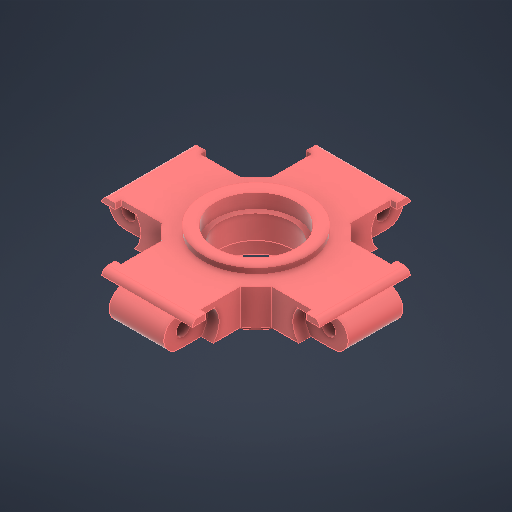
# Autodesk Inventor part: SujeccionHelices
Saved by Autodesk Inventor 2026.1 (Build 301233000, 233)
## iProperties
Created: 2025-11-10
Part Number: SujeccionHelices
Material: PLA
Document SubType Name: Modeling
Designer: vickh
Density: 1.3 g/cm^3
Appearance: Suave - Rojo
Mass: 57.6997 g
Surface Area: 138.679 cm^2
Volume: 44.3844 cm^3
Author: vickh
## iProperties of the stored document SujeccionHelices_3DPrint.ipt
Created: 2025-11-17
Part Number: SujeccionHelices_3DPrint
Material: Genérico
Document SubType Name: Modeling
Designer: usuario
Density: 1 g/cm^3
Appearance: Valor por defecto
Author: usuario
Autodesk Inventor part; units mm, degrees
ref_plane "YZ Plane" through (0, 0, 0) normal (1, 0, 0) x (0, 1, 0)
ref_plane "XZ Plane" through (0, 0, 0) normal (0, 1, 0) x (-1, 0, 0)
ref_plane "XY Plane" through (0, 0, 0) normal (0, 0, 1) x (1, 0, 0)
sketch "Boceto27" plane through (0, 0, 0) normal (0, 1, 0) x (-1, 0, 0)
  line L0 (13.15, -40) -> (-13.15, -40)
  line L1 (-13.15, 40) -> (13.15, 40)
  line L2 (13.15, 40) -> (-13.15, -40) construction
  line L3 (13.15, -40) -> (-13.15, 40) construction
  line L4 (-40, 13.15) -> (-40, -13.15)
  line L5 (40, -13.15) -> (40, 13.15)
  line L6 (-40, 13.15) -> (40, -13.15) construction
  line L7 (-40, -13.15) -> (40, 13.15) construction
  line L8 (40, 13.15) -> (18.2573, 13.15)
  line L9 (13.15, 40) -> (13.15, 18.2573)
  line L10 (-13.15, 18.2573) -> (-13.15, 40)
  line L11 (13.15, -18.2573) -> (13.15, -40)
  line L12 (-40, -13.15) -> (-18.2573, -13.15)
  line L13 (18.2573, -13.15) -> (40, -13.15)
  line L14 (-18.2573, 13.15) -> (-40, 13.15)
  line L15 (-13.15, -40) -> (-13.15, -18.2573)
  arc A0 (13.15, -18.2573) -> (18.2573, -13.15) centre (0, 0) ccw
  arc A1 (18.2573, 13.15) -> (13.15, 18.2573) centre (0, 0) ccw
  arc A2 (-13.15, 18.2573) -> (-18.2573, 13.15) centre (0, 0) ccw
  arc A3 (-18.2573, -13.15) -> (-13.15, -18.2573) centre (0, 0) ccw
  point P0 (13.15, -29.1286)
  dimension "d134" = 80
  dimension "d135" = 26.3
  dimension "d136" = 26.3
  dimension "d137" = 80
  dimension "d138" = 22.5
  dimension "d139" = 22.5
  dimension "d140" = 22.5
  dimension "d141" = 22.5
  constraints: 32 end point, 12 parallel, 8 point on circle, 5 midpoint, 4 centre point, 4 perpendicular, 3 collinear, 2 vertical, 1 coincident, 1 point on line
  measures "d134" distance of L1.end L0.start
  measures "d135" distance of L0.start L0.end
  measures "d136" distance of L4.start L4.end
  measures "d137" distance of L5.start L4.end
  measures "d138" radius of A1
  measures "d139" radius of A0
  measures "d140" radius of A3
  measures "d141" radius of A2
extrude "Extrusión24" add sketch "Boceto27" along normal blind 18
sketch "Boceto28" plane through (0, 18, 0) normal (0, 1, 0) x (1, 0, 0)
  circle A0 centre (0, 0) radius 12
  circle A1 centre (0, 0) radius 13.5
  dimension "d145" = 24
  dimension "d146" = 27
  constraints: 2 centre point, 2 coincident
  measures "d145" diameter of A0
  measures "d146" diameter of A1
extrude "Extrusión25" cut sketch "Boceto28" against normal up to next contours A0
extrude "Extrusión26" cut sketch "Boceto28" against normal blind 5
sketch "Boceto29" plane through (0, 0, 0) normal (0, -1, 0) x (1, 0, 0)
  circle A0 centre (0, 0) radius 13.5
  dimension "d151" = 27
  constraints: 1 centre point, 1 coincident
  measures "d151" diameter of A0
extrude "Extrusión27" cut sketch "Boceto29" against normal blind 5
sketch "Boceto45" plane through (0, 18, 0) normal (0, 1, 0) x (1, 0, 0)
  point P0 (0, 0)
sketch "Boceto46" plane through (0, 18, 0) normal (0, 1, 0) x (1, 0, 0)
  circle A0 centre (0, 0) radius 17.5
  circle A1 centre (0, 0) radius 13.5 projected
  line L0 (-18.2573, 13.15) -> (-40, 13.15) projected
  line L1 (-40, 13.15) -> (-40, -13.15) projected
  line L2 (-40, -13.15) -> (-18.2573, -13.15) projected
  arc A2 (-18.2573, -13.15) -> (-13.15, -18.2573) centre (0, 0) ccw projected
  line L3 (-13.15, -18.2573) -> (-13.15, -40) projected
  line L4 (-13.15, -40) -> (13.15, -40) projected
  line L5 (13.15, -40) -> (13.15, -18.2573) projected
  arc A3 (13.15, -18.2573) -> (18.2573, -13.15) centre (0, 0) ccw projected
  line L6 (18.2573, -13.15) -> (40, -13.15) projected
  line L7 (40, -13.15) -> (40, 13.15) projected
  line L8 (40, 13.15) -> (18.2573, 13.15) projected
  arc A4 (18.2573, 13.15) -> (13.15, 18.2573) centre (0, 0) ccw projected
  line L9 (13.15, 18.2573) -> (13.15, 40) projected
  line L10 (13.15, 40) -> (-13.15, 40) projected
  line L11 (-13.15, 40) -> (-13.15, 18.2573) projected
  arc A5 (-13.15, 18.2573) -> (-18.2573, 13.15) centre (0, 0) ccw projected
  dimension "d192" = 35
  constraints: 1 centre point, 1 coincident
  measures "d192" diameter of A0
extrude "Extrusión36" cut sketch "Boceto46" against normal blind 4 contours A5 L11 L10 L9 A4 L8 L7 L6 A3 L5 L4 L3 A2 L2 L1 L0
sketch "Boceto47" plane through (0, 0, 0) normal (0, -1, 0) x (1, 0, 0)
  circle A0 centre (0, 0) radius 12 projected
  circle A1 centre (0, 0) radius 17.5
  circle A2 centre (0, 0) radius 13.5 projected
  line L0 (-18.2573, -13.15) -> (-40, -13.15) projected
  arc A3 (-18.2573, -13.15) -> (-13.15, -18.2573) centre (0, 0) ccw projected
  line L1 (-13.15, -40) -> (-13.15, -18.2573) projected
  line L2 (13.15, -40) -> (-13.15, -40) projected
  line L3 (13.15, -18.2573) -> (13.15, -40) projected
  arc A4 (13.15, -18.2573) -> (18.2573, -13.15) centre (0, 0) ccw projected
  line L4 (40, -13.15) -> (18.2573, -13.15) projected
  line L5 (40, 13.15) -> (40, -13.15) projected
  line L6 (18.2573, 13.15) -> (40, 13.15) projected
  arc A5 (18.2573, 13.15) -> (13.15, 18.2573) centre (0, 0) ccw projected
  line L7 (13.15, 40) -> (13.15, 18.2573) projected
  line L8 (-13.15, 40) -> (13.15, 40) projected
  line L9 (-13.15, 18.2573) -> (-13.15, 40) projected
  arc A6 (-13.15, 18.2573) -> (-18.2573, 13.15) centre (0, 0) ccw projected
  line L10 (-40, 13.15) -> (-18.2573, 13.15) projected
  line L11 (-40, -13.15) -> (-40, 13.15) projected
  dimension "d195" = 35
  constraints: 1 centre point, 1 coincident
  measures "d195" diameter of A1
extrude "Extrusión37" cut sketch "Boceto47" against normal blind 4 contours L0 L11 L10 A6 L9 L8 L7 A5 L6 L5 L4 A4 L3 L2 L1 A3
sketch "Boceto30" plane through (-18.2573, 0, -13.15) normal (0, 0, -1) x (-1, 0, 0)
  line L0 (21.7427, 18) -> (0, 18) projected
  line L1 (21.7427, 0) -> (21.7427, 18) projected
  line L2 (0, 18) -> (21.7427, 0) construction
  line L3 (0, 0) -> (21.7427, 0) construction
  line L4 (0, 0) -> (21.7427, 18) construction
  circle A0 centre (15.2427, 9.3) radius 2.25
  line L5 (0, 18) -> (21.7427, 18) projected
  line L6 (10.8714, 18) -> (10.8714, 0) construction
  line L7 (0, 4) -> (21.7427, 4) projected
  line L8 (0, 4) -> (0, 14) construction
  line L9 (0, 9) -> (21.7427, 9) construction
  point P0 (-18.2573, 0)
  point P1 (10.8714, 9)
  point P2 (10.8714, 9)
  dimension "d159" = 4.5
  dimension "d198" = 6.5
  dimension "d238" = 0.3
  constraints: 8 end point, 6 midpoint, 1 centre point
  measures "d159" diameter of A0
  measures "d198" distance from line of L1 A0.centre
  measures "d238" distance from line of L9 A0.centre
sketch "Boceto32" plane through (-13.15, 0, -40) normal (-1, 0, 0) x (0, 0, 1)
  line L0 (0, 0) -> (0, 18) projected
  line L1 (21.7427, 0) -> (21.7427, 18) projected
  line L2 (0, 18) -> (21.7427, 0) construction
  line L3 (21.7427, 0) -> (0, 0) construction
  line L4 (0, 0) -> (21.7427, 18) construction
  point P0 (40, 0)
  point P1 (10.8714, 9)
  constraints: 4 end point, 1 midpoint
sketch "Boceto33" plane through (0, 18, 0) normal (0, 1, 0) x (1, 0, 0)
  line L0 (29.1286, -29.1286) -> (-29.1286, -29.1286)
  line L1 (-29.1286, -29.1286) -> (-29.1286, 29.1286)
  line L2 (-29.1286, 29.1286) -> (29.1286, 29.1286)
  line L3 (29.1286, 29.1286) -> (29.1286, -29.1286)
  line L4 (29.1286, -29.1286) -> (-29.1286, 29.1286) construction
  line L5 (-29.1286, -29.1286) -> (29.1286, 29.1286) construction
  line L6 (-18.2573, 13.15) -> (-40, 13.15) projected
  line L7 (-13.15, 40) -> (-13.15, 18.2573) projected
  point P0 (0, 0)
  point P1 (-29.1286, 13.15)
  point P2 (-13.15, 29.1286)
  point P3 (-13.15, 29.1286)
  constraints: 12 end point, 4 midpoint, 2 parallel, 2 point on line, 1 horizontal, 1 perpendicular
sweep "Barrido2" cut profiles "Boceto30" path "Boceto33" path curves L1 L0 L3 L2
sketch "Boceto48" plane through (13.15, 14, -18.2573) normal (1, 0, 0) x (0, 0, -1)
  circle A0 centre (15.2427, -4.7) radius 2.25 projected
  circle A1 centre (15.2427, -4.7) radius 8
  circle A2 centre (-51.7573, -4.7) radius 2.25 projected
  circle A3 centre (-51.7573, -4.7) radius 8
  line L0 (-31.4073, -6.95) -> (-31.4073, -2.45) projected
  point P0 (-18.2573, -14)
  dimension "d200" = 16
  dimension "d203" = 16
  constraints: 2 centre point, 2 coincident
  measures "d200" diameter of A1
  measures "d203" diameter of A3
sketch "Boceto49" plane through (18.2573, 14, 13.15) normal (0, 0, 1) x (1, 0, 0)
  circle A0 centre (15.2427, -4.7) radius 2.25 projected
  circle A1 centre (-51.7573, -4.7) radius 2.25 projected
  circle A2 centre (15.2427, -4.7) radius 8
  circle A3 centre (-51.7573, -4.7) radius 8
  point P0 (-18.2573, -14)
  dimension "d204" = 16
  dimension "d205" = 16
  constraints: 2 centre point, 2 coincident
  measures "d204" diameter of A2
  measures "d205" diameter of A3
sketch "Boceto50" plane through (-13.15, 14, -40) normal (-1, 0, 0) x (0, 0, 1)
  circle A0 centre (6.5, -4.7) radius 2.25 projected
  circle A1 centre (6.5, -4.7) radius 8
  circle A2 centre (73.5, -4.7) radius 2.25 projected
  circle A3 centre (73.5, -4.7) radius 8
  point P0 (40, -14)
  dimension "d206" = 16
  dimension "d207" = 16
  constraints: 2 centre point, 2 coincident
  measures "d206" diameter of A1
  measures "d207" diameter of A3
sketch "Boceto52" plane through (40, 14, -13.15) normal (0, 0, -1) x (-1, 0, 0)
  circle A0 centre (6.5, -4.7) radius 2.25 projected
  circle A1 centre (73.5, -4.7) radius 2.25 projected
  circle A2 centre (6.5, -4.7) radius 8
  circle A3 centre (73.5, -4.7) radius 8
  point P0 (40, -14)
  dimension "d208" = 16
  dimension "d209" = 16
  constraints: 2 centre point, 2 coincident
  measures "d208" diameter of A2
  measures "d209" diameter of A3
extrude "Extrusión39" cut sketch "Boceto52" against normal blind 4 contours A1 | A2 | A3
extrude "Extrusión40" cut sketch "Boceto48" against normal blind 4 contours A0 | A1 | A2 | A3
extrude "Extrusión41" cut sketch "Boceto50" against normal blind 4 contours A0 | A1 | A2 | A3
extrude "Extrusión42" cut sketch "Boceto49" against normal blind 4 contours A0 | A1 | A2 | A3
sketch "Boceto53" plane through (0, 4, 0) normal (0, -1, 0) x (1, 0, 0)
  circle A0 centre (0, 0) radius 17.5 projected
  line L0 (39.4925, 13.15) -> (39.4925, 9.15) projected
  line L1 (39.4925, 9.15) -> (27.5075, 9.15) projected
  line L2 (27.5075, 9.15) -> (27.5075, 13.15) projected
  line L3 (18.2573, 13.15) -> (27.5075, 13.15) projected
  arc A1 (18.2573, 13.15) -> (13.15, 18.2573) centre (0, 0) ccw projected
  line L4 (13.15, 27.5075) -> (13.15, 18.2573) projected
  line L5 (13.15, 27.5075) -> (9.15, 27.5075) projected
  line L6 (9.15, 27.5075) -> (9.15, 39.4925) projected
  line L7 (9.15, 39.4925) -> (13.15, 39.4925) projected
  line L8 (13.15, 40) -> (13.15, 39.4925) projected
  line L9 (-13.15, 40) -> (13.15, 40) projected
  line L10 (-13.15, 39.4925) -> (-13.15, 40) projected
  line L11 (-13.15, 39.4925) -> (-9.15, 39.4925) projected
  line L12 (-9.15, 39.4925) -> (-9.15, 27.5075) projected
  line L13 (-9.15, 27.5075) -> (-13.15, 27.5075) projected
  line L14 (-13.15, 18.2573) -> (-13.15, 27.5075) projected
  arc A2 (-13.15, 18.2573) -> (-18.2573, 13.15) centre (0, 0) ccw projected
  line L15 (-27.5075, 13.15) -> (-18.2573, 13.15) projected
  line L16 (-27.5075, 13.15) -> (-27.5075, 9.15) projected
  line L17 (-27.5075, 9.15) -> (-39.4925, 9.15) projected
  line L18 (-39.4925, 9.15) -> (-39.4925, 13.15) projected
  line L19 (-40, 13.15) -> (-39.4925, 13.15) projected
  line L20 (-40, -13.15) -> (-40, 13.15) projected
  line L21 (-39.4925, -13.15) -> (-40, -13.15) projected
  line L22 (-39.4925, -13.15) -> (-39.4925, -9.15) projected
  line L23 (-39.4925, -9.15) -> (-27.5075, -9.15) projected
  line L24 (-27.5075, -9.15) -> (-27.5075, -13.15) projected
  line L25 (-18.2573, -13.15) -> (-27.5075, -13.15) projected
  arc A3 (-18.2573, -13.15) -> (-13.15, -18.2573) centre (0, 0) ccw projected
  line L26 (-13.15, -27.5075) -> (-13.15, -18.2573) projected
  line L27 (-13.15, -27.5075) -> (-9.15, -27.5075) projected
  line L28 (-9.15, -27.5075) -> (-9.15, -39.4925) projected
  line L29 (-9.15, -39.4925) -> (-13.15, -39.4925) projected
  line L30 (-13.15, -40) -> (-13.15, -39.4925) projected
  line L31 (13.15, -40) -> (-13.15, -40) projected
  line L32 (13.15, -39.4925) -> (13.15, -40) projected
  line L33 (13.15, -39.4925) -> (9.15, -39.4925) projected
  line L34 (9.15, -39.4925) -> (9.15, -27.5075) projected
  line L35 (9.15, -27.5075) -> (13.15, -27.5075) projected
  line L36 (13.15, -18.2573) -> (13.15, -27.5075) projected
  arc A4 (13.15, -18.2573) -> (18.2573, -13.15) centre (0, 0) ccw projected
  line L37 (27.5075, -13.15) -> (18.2573, -13.15) projected
  line L38 (27.5075, -13.15) -> (27.5075, -9.15) projected
  line L39 (27.5075, -9.15) -> (39.4925, -9.15) projected
  line L40 (39.4925, -9.15) -> (39.4925, -13.15) projected
  line L41 (40, -13.15) -> (39.4925, -13.15) projected
  line L42 (40, 13.15) -> (40, -13.15) projected
  line L43 (39.4925, 13.15) -> (40, 13.15) projected
  line L44 (-13.15, 33.7538) -> (13.15, 33.7538)
  line L45 (-9.15, 35.75) -> (-9.15, 31.25) projected
  line L46 (-9.15, 27.0262) -> (-9.15, 39.9738) projected
  line L47 (-13.15, 40) -> (13.15, 27.5075) construction
  circle A5 centre (0, 0) radius 17.5 construction
  line L48 (-13.15, 33.7538) -> (-13.15, 40)
  line L49 (13.15, 33.7538) -> (13.15, 40)
  line L50 (-9.15, 39.4925) -> (-9.15, 27.5075) projected
  line L51 (-9.15, 33.7538) -> (-9.15, 40)
  line L52 (9.15, 33.7538) -> (9.15, 40)
  line L53 (-33.7538, -13.15) -> (-33.7538, 13.15)
  line L54 (-33.7538, 13.15) -> (-40, 13.15)
  line L55 (-33.7538, 9.15) -> (-40, 9.15)
  line L56 (-33.7538, -9.15) -> (-40, -9.15)
  line L57 (-33.7538, -13.15) -> (-40, -13.15)
  line L58 (13.15, -33.7538) -> (-13.15, -33.7538)
  line L59 (-13.15, -33.7538) -> (-13.15, -40)
  line L60 (-9.15, -33.7538) -> (-9.15, -40)
  line L61 (9.15, -33.7538) -> (9.15, -40)
  line L62 (13.15, -33.7538) -> (13.15, -40)
  line L63 (33.7538, 13.15) -> (33.7538, -13.15)
  line L64 (33.7538, -13.15) -> (40, -13.15)
  line L65 (33.7538, -9.15) -> (40, -9.15)
  line L66 (33.7538, 9.15) -> (40, 9.15)
  line L67 (33.7538, 13.15) -> (40, 13.15)
  point P0 (0, 33.7538)
  point P1 (-39.4925, 9.15)
  point P2 (-39.4925, 13.15)
  point P3 (-39.4925, -13.15)
  point P4 (-33.7538, 0)
  point P5 (-39.4925, -9.15)
  point P6 (-35.75, -9.15)
  point P7 (-39.9738, -9.15)
  point P8 (-9.15, -39.4925)
  point P9 (-13.15, -39.4925)
  point P10 (13.15, -39.4925)
  point P11 (0, -33.7538)
  point P12 (9.15, -39.4925)
  point P13 (9.15, -35.75)
  point P14 (9.15, -39.9738)
  point P15 (39.4925, -9.15)
  point P16 (39.4925, -13.15)
  point P17 (39.4925, 13.15)
  point P18 (33.7538, 0)
  point P19 (39.4925, 9.15)
  point P20 (35.75, 9.15)
  point P21 (39.9738, 9.15)
  point P22 (33.7538, -9.15)
  point P23 (33.7538, 9.15)
  point P24 (9.15, -33.7538)
  point P25 (-33.7538, -9.15)
  point P26 (-33.7538, 9.15)
  point P27 (-9.15, 33.7538)
  dimension "d220" = 360
  constraints: 42 end point, 14 point on line, 2 midpoint, 1 horizontal, 1 parallel, 1 vertical, 81 other
extrude "Extrusión43" cut sketch "Boceto53" against normal blind 16 contours L43 L42 L66 L0 | L0 L1 L63 L67 | L39 L40 L64 L63 | L42 L41 L40 L65 | L6 L7 L49 L44 | L52 L9 L8 L7 | L44 L48 L11 L12 | L58 L62 L33 L34 | L33 L32 L31 L61 | L28 L29 L59 L58 | L51 L46 L11 L10 L9 | L60 L31 L30 L29 | L17 L18 L54 L53 | L53 L57 L22 L23 | L55 L20 L19 L18 | L22 L21 L20 L56
fillet "Empalme9" radius 5 8 edges at (-40, 14, 0) (-40, 4, 0) (0, 14, 40) (0, 4, 40) (40, 14, 0) (40, 4, 0) (0, 14, -40) (0, 4, -40)
sketch "Boceto54" plane through (0, 14, 0) normal (0, 1, 0) x (1, 0, 0)
  line L0 (-9.15, 35) -> (9.15, 35) projected
  line L1 (-9.15, 35) -> (-9.15, 27.0262) projected
  line L2 (-9.15, 27.0262) -> (-13.15, 27.0262) projected
  line L3 (-13.15, 18.2573) -> (-13.15, 27.0262) projected
  arc A0 (-13.15, 18.2573) -> (-18.2573, 13.15) centre (0, 0) ccw projected
  line L4 (-27.0262, 13.15) -> (-18.2573, 13.15) projected
  line L5 (-27.0262, 13.15) -> (-27.0262, 9.15) projected
  line L6 (-27.0262, 9.15) -> (-35, 9.15) projected
  line L7 (-35, -9.15) -> (-35, 9.15) projected
  line L8 (-35, -9.15) -> (-27.0262, -9.15) projected
  line L9 (-27.0262, -9.15) -> (-27.0262, -13.15) projected
  line L10 (-18.2573, -13.15) -> (-27.0262, -13.15) projected
  arc A1 (-18.2573, -13.15) -> (-13.15, -18.2573) centre (0, 0) ccw projected
  line L11 (-13.15, -27.0262) -> (-13.15, -18.2573) projected
  line L12 (-13.15, -27.0262) -> (-9.15, -27.0262) projected
  line L13 (-9.15, -27.0262) -> (-9.15, -35) projected
  line L14 (9.15, -35) -> (-9.15, -35) projected
  line L15 (9.15, -35) -> (9.15, -27.0262) projected
  line L16 (9.15, -27.0262) -> (13.15, -27.0262) projected
  line L17 (13.15, -18.2573) -> (13.15, -27.0262) projected
  arc A2 (13.15, -18.2573) -> (18.2573, -13.15) centre (0, 0) ccw projected
  line L18 (27.0262, -13.15) -> (18.2573, -13.15) projected
  line L19 (27.0262, -13.15) -> (27.0262, -9.15) projected
  line L20 (27.0262, -9.15) -> (35, -9.15) projected
  line L21 (35, 9.15) -> (35, -9.15) projected
  line L22 (35, 9.15) -> (27.0262, 9.15) projected
  line L23 (27.0262, 9.15) -> (27.0262, 13.15) projected
  line L24 (18.2573, 13.15) -> (27.0262, 13.15) projected
  arc A3 (18.2573, 13.15) -> (13.15, 18.2573) centre (0, 0) ccw projected
  line L25 (13.15, 27.0262) -> (13.15, 18.2573) projected
  line L26 (13.15, 27.0262) -> (9.15, 27.0262) projected
  line L27 (9.15, 27.0262) -> (9.15, 35) projected
  circle A4 centre (0, 0) radius 17.5 projected
  line L28 (9.15, 40) -> (9.15, 35) projected
  line L29 (-9.15, 35) -> (-9.15, 40) projected
  line L30 (-9.15, 40) -> (9.15, 40) projected
  line L31 (40, -9.15) -> (35, -9.15) projected
  line L32 (35, 9.15) -> (40, 9.15) projected
  line L33 (40, 9.15) -> (40, -9.15) projected
  line L34 (9.15, -40) -> (-9.15, -40) projected
  line L35 (9.15, -35) -> (9.15, -40) projected
  line L36 (-9.15, -40) -> (-9.15, -35) projected
  line L37 (-35, -9.15) -> (-40, -9.15) projected
  line L38 (-40, 9.15) -> (-35, 9.15) projected
  line L39 (-40, -9.15) -> (-40, 9.15) projected
  line L40 (-15.15, 32.0262) -> (15.15, 32.0262)
  line L41 (15.15, 32.0262) -> (15.15, 36.5)
  line L42 (15.15, 36.5) -> (-15.15, 36.5)
  line L43 (-15.15, 36.5) -> (-15.15, 32.0262)
  line L44 (-13.15, 27.0262) -> (-13.15, 32.0262)
  line L45 (9.15, 27.5075) -> (13.15, 27.5075) projected
  line L46 (13.15, 27.0262) -> (13.15, 32.0262)
  line L47 (-27.0262, -13.15) -> (-32.0262, -13.15)
  line L48 (-32.0262, -15.15) -> (-32.0262, 15.15)
  line L49 (-36.5, -15.15) -> (-32.0262, -15.15)
  line L50 (-36.5, 15.15) -> (-36.5, -15.15)
  line L51 (-27.0262, 13.15) -> (-32.0262, 13.15)
  line L52 (-32.0262, 15.15) -> (-36.5, 15.15)
  line L53 (13.15, -27.0262) -> (13.15, -32.0262)
  line L54 (15.15, -32.0262) -> (-15.15, -32.0262)
  line L55 (15.15, -36.5) -> (15.15, -32.0262)
  line L56 (-15.15, -36.5) -> (15.15, -36.5)
  line L57 (-13.15, -27.0262) -> (-13.15, -32.0262)
  line L58 (-15.15, -32.0262) -> (-15.15, -36.5)
  line L59 (27.0262, 13.15) -> (32.0262, 13.15)
  line L60 (32.0262, 15.15) -> (32.0262, -15.15)
  line L61 (36.5, 15.15) -> (32.0262, 15.15)
  line L62 (36.5, -15.15) -> (36.5, 15.15)
  line L63 (27.0262, -13.15) -> (32.0262, -13.15)
  line L64 (32.0262, -15.15) -> (36.5, -15.15)
  point P0 (15.15, 34.2631)
  point P1 (-15.15, 34.2631)
  point P2 (-9.15, 31.0131)
  point P3 (-35, 9.15)
  point P4 (-35, -9.15)
  point P5 (-27.0262, -9.15)
  point P6 (-27.0262, 9.15)
  point P7 (-31.0131, -9.15)
  point P8 (-34.2631, -15.15)
  point P9 (-34.2631, 15.15)
  point P10 (-9.15, -35)
  point P11 (9.15, -35)
  point P12 (9.15, -27.0262)
  point P13 (-9.15, -27.0262)
  point P14 (9.15, -31.0131)
  point P15 (15.15, -34.2631)
  point P16 (-15.15, -34.2631)
  point P17 (35, -9.15)
  point P18 (35, 9.15)
  point P19 (27.0262, 9.15)
  point P20 (27.0262, -9.15)
  point P21 (31.0131, 9.15)
  point P22 (34.2631, 15.15)
  point P23 (34.2631, -15.15)
  dimension "d226" = 6
  dimension "d227" = 6
  dimension "d230" = 5
  dimension "d231" = 1.5
  dimension "d234" = 360
  constraints: 48 end point, 8 point on line, 3 midpoint, 3 perpendicular, 2 parallel, 1 horizontal, 85 other
  measures "d226" distance from line of point (15.15, 34.263) L27
  measures "d227" horizontal distance of point (-15.15, 34.263) point (-9.15, 31.013)
  measures "d230" distance between parallel lines of L40 L2
  measures "d231" distance between parallel lines of L42 L0
extrude "Extrusión44" add sketch "Boceto54" along normal blind 2 contours L29 L42 L28 L0 | L0 L27 L40 L1 | L1 L40 L43 L42 L29 | L28 L42 L41 L40 L27 | L40 L27 L26 L25 A3 L24 L23 L22 L60 L20 L19 L18 A2 L17 L16 L15 L54 L13 L12 L11 A1 L10 L9 L8 L48 L6 L5 L4 A0 L3 L2 L1 | L1 L2 L44 L40 | L40 L46 L45 L27 | L45 L46 L26 L27 | L5 L6 L48 L51 | L48 L6 L38 L50 L52 | L59 L60 L22 L23 | L48 L8 L7 L6 | L60 L61 L62 L32 L22 | L7 L37 L50 L38 | L48 L49 L50 L37 L8 | L8 L9 L47 L48 | L22 L21 L20 L60 | L32 L62 L31 L21 | L60 L63 L19 L20 | L20 L31 L62 L64 L60 | L12 L13 L54 L57 | L54 L13 L36 L56 L58 | L53 L54 L15 L16 | L54 L15 L14 L13 | L54 L55 L56 L35 L15 | L14 L35 L56 L36
fillet "Empalme10" radius 2 4 edges at (0, 16, -36.5) (36.5, 16, 0) (0, 16, 36.5) (-36.5, 16, 0)
